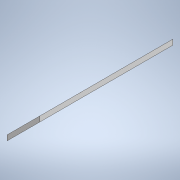
# Autodesk Inventor part: Part14
Saved by Autodesk Inventor 2022 (Build 260153000, 153)
## iProperties
Created: 2022-12-09
Part Number: Part14
Material: Generic
Document SubType Name: Modeling
Designer: Kamil
Density: 1 g/cm^3
Appearance: Default
Author: Kamil
Autodesk Inventor part; units mm, degrees
ref_plane "YZ Plane" through (0, 0, 0) normal (1, 0, 0) x (0, 1, 0)
ref_plane "XZ Plane" through (0, 0, 0) normal (0, 1, 0) x (-1, 0, 0)
ref_plane "XY Plane" through (0, 0, 0) normal (0, 0, 1) x (1, 0, 0)
sketch "Sketch1" plane through (0, 0, 0) normal (0, 0, 1) x (1, 0, 0)
  line L0 (0, 57.4166) -> (-5, 46.6664) projected
  line L1 (-5, 42.7444) -> (-5, 46.6664) projected
  line L2 (-5, 42.7444) -> (-29.7, 18.0444) projected
  line L3 (-29.7, 18.0444) -> (-29.7, -5.3095) projected
  arc A0 (-5, 0) -> (-29.7, -5.3095) centre (-13.6, -20.1) ccw projected
  line L4 (0, 0) -> (-5, 0) projected
  line L5 (0, 0) -> (0, 57.4166) projected
  line L6 (-29.7, 18.0444) -> (-29.7, 25.3757)
  line L7 (-5, 46.6664) -> (-29.7, 21.9664)
  constraints: 4 end point, 1 point on line, 1 vertical
extrude "Extrusion1" add sketch "Sketch1" against normal blind 100 contours L1 L2 L6 L7
body "Solid1"
